Autodesk Fusion 360 part; units mm, degrees
note: some values were not read from the file. Set by a fixed rule: which face or edge a step refers to.
(part 2 of 2)
sketch "Sketch1 (3)" plane through (-20, 0, 0) normal (-1, 0, 0) x (0, -1, 0) in component "Brazo_superior"
  spline S0 degree 5 poles (211.9586, 262.8712) (213.9, 262.5) (215, 260) (215, 257) (212.5679, 252.5298) (212.2678, 249.9329) (212.5261, 247.5635) (214.6128, 241.6791) (217, 240) (218.5775, 235.2522) (220, 231) (221, 229) (220.5807, 226.196) (217.5759, 223.692) (213.5278, 221.7305) (209.5631, 220.0194) (204.555, 219.2265) (203, 220) (201.592, 223.2329) (202, 228) (201.9676, 233.4159) (203.5534, 240.5523) (204.8472, 246.5619) (206.5583, 254.533) (209.5, 263.2) (210.4715, 262.8927) (211.9586, 262.8712) knots 0 0 0 0 0 0 0.045455 0.090909 0.136364 0.181818 0.227273 0.272727 0.318182 0.363636 0.409091 0.454545 0.5 0.545455 0.590909 0.636364 0.681818 0.727273 0.772727 0.818182 0.863636 0.909091 0.954545 1 1 1 1 1 1
  spline S1 degree 5 poles (261, 320) (260.7774, 319.9589) (260.296, 319.9643) (259.4625, 320.2428) (258.1325, 321.1584) (256.169, 323.121) (254.0011, 325.7467) (251.739, 328.8478) (249.4883, 332.2331) (247.3274, 335.7454) (245.3055, 339.2672) (243.4488, 342.7117) (241.7644, 346.0192) (240.2451, 349.1514) (238.8737, 352.0857) (237.6281, 354.8109) (236.4846, 357.3206) (235.4258, 359.6112) (234.4564, 361.6897) (233.6206, 363.5797) (233.0136, 365.3267) (232.8084, 367.0089) (233.2246, 368.7247) (234.4249, 370.5487) (236.4437, 372.5039) (239.0716, 374.5107) (241.9507, 376.4378) (244.6888, 378.1513) (247.0272, 379.6106) (248.853, 380.8435) (250.59, 382.2095) (252.6141, 383.9228) (254.5082, 385.553) (255.9404, 386.771) (256.8623, 387.5494) (258.3073, 388.9023) (260.3731, 390.8134) (262.725, 392.7952) (264.822, 394.1558) (266.2188, 394.3429) (266.8921, 393.3204) (267.1118, 391.4187) (267.1481, 388.996) (267.134, 386.2763) (267.1221, 383.4019) (267.1026, 380.4443) (267.0374, 377.4316) (266.8857, 374.368) (266.6365, 371.2585) (266.3041, 368.1107) (265.9189, 364.9337) (265.5197, 361.7382) (265.1452, 358.5361) (264.827, 355.3399) (264.5793, 352.1629) (264.3983, 349.0181) (264.2687, 345.918) (264.1682, 342.8735) (264.0738, 339.8935) (263.9654, 336.984) (263.8335, 334.147) (263.6787, 331.3832) (263.501, 328.7082) (263.2907, 326.1645) (263.0185, 323.8353) (262.6258, 321.8583) (262.1382, 320.7217) (261.6314, 320.2111) (261.2226, 320.0411) (261, 320) knots 0 0 0 0 0 0 0.01538462 0.03076923 0.04615385 0.06153846 0.07692308 0.09230769 0.10769231 0.12307692 0.13846154 0.15384615 0.16923077 0.18461538 0.2 0.21538462 0.23076923 0.24615385 0.26153846 0.27692308 0.29230769 0.30769231 0.32307692 0.33846154 0.35384615 0.36923077 0.38461538 0.4 0.41538462 0.43076923 0.44615385 0.46153846 0.47692308 0.49230769 0.50769231 0.52307692 0.53846154 0.55384615 0.56923077 0.58461538 0.6 0.61538462 0.63076923 0.64615385 0.66153846 0.67692308 0.69230769 0.70769231 0.72307692 0.73846154 0.75384615 0.76923077 0.78461538 0.8 0.81538462 0.83076923 0.84615385 0.86153846 0.87692308 0.89230769 0.90769231 0.92307692 0.93846154 0.95384615 0.96923077 0.98461538 1 1 1 1 1 1
  spline S2 degree 5 poles (213.7541, 291.5012) (213.7836, 292.1337) (213.9165, 293.5506) (214.3357, 296.1342) (215.3059, 300.4504) (217.0551, 306.9808) (219.1416, 314.1905) (221.3444, 321.5493) (223.447, 328.5165) (225.2663, 334.6064) (226.678, 339.4493) (227.6481, 342.8655) (228.2526, 344.9081) (228.7265, 345.9852) (229.415, 346.7173) (230.5211, 347.2402) (231.9417, 346.7519) (233.4976, 344.3536) (235.4615, 340.7393) (237.9174, 336.5993) (240.7362, 332.3678) (243.6759, 328.3703) (246.4235, 324.7873) (248.6618, 321.698) (250.1239, 319.0883) (250.6571, 316.8737) (250.2721, 314.9163) (249.0801, 313.0601) (247.2465, 311.16) (244.9297, 309.119) (242.2549, 306.9017) (239.3271, 304.5172) (236.2338, 302.0107) (233.052, 299.4513) (229.8531, 296.9221) (226.7094, 294.5083) (223.6983, 292.2901) (220.9029, 290.3618) (218.4131, 288.8445) (216.3267, 287.9051) (214.7483, 287.7655) (213.986, 288.5405) (213.7397, 289.7559) (213.7247, 290.8688) (213.7541, 291.5012) knots 0 0 0 0 0 0 0.025 0.05 0.075 0.1 0.125 0.15 0.175 0.2 0.225 0.25 0.275 0.3 0.325 0.35 0.375 0.4 0.425 0.45 0.475 0.5 0.525 0.55 0.575 0.6 0.625 0.65 0.675 0.7 0.725 0.75 0.775 0.8 0.825 0.85 0.875 0.9 0.925 0.95 0.975 1 1 1 1 1 1
  spline S3 degree 5 poles (213.9418, 208.154) (213.814, 207.7824) (213.413, 207.0453) (212.3788, 205.9701) (210.2085, 204.6435) (206.5692, 203.2643) (202.5179, 202.2474) (198.6058, 201.6547) (195.339, 201.5236) (193.0886, 201.8616) (192.0173, 202.6437) (191.9595, 203.8037) (192.5257, 205.2474) (193.2802, 206.8702) (193.9221, 208.5769) (194.3624, 210.2884) (194.6519, 211.9313) (194.9497, 213.4312) (195.4767, 214.7047) (196.4747, 215.6545) (198.1353, 216.19) (200.5393, 216.2433) (203.5777, 215.7898) (206.9221, 214.8595) (210.1263, 213.5214) (212.7024, 211.8749) (213.9048, 210.4054) (214.1797, 209.275) (214.0696, 208.5256) (213.9418, 208.154) knots -1 -1 -1 -1 -1 -1 -0.96 -0.92 -0.88 -0.84 -0.8 -0.76 -0.72 -0.68 -0.64 -0.6 -0.56 -0.52 -0.48 -0.44 -0.4 -0.36 -0.32 -0.28 -0.24 -0.2 -0.16 -0.12 -0.08 -0.04 0 0 0 0 0 0
  spline S4 degree 3 poles (231.4249, 227.1643) (225.7976, 239.2027) (227.1439, 245.9013) (243.6188, 239.3572) knots -0.949588 -0.949588 -0.949588 -0.949588 -0.175444 -0.175444 -0.175444 -0.175444
  arc A0 (243.9542, 237.7182) -> (243.6188, 239.3572) centre (243.2497, 238.4278) ccw
  line L0 (243.9542, 237.7182) -> (233.0354, 226.8781)
  arc A1 (231.4249, 227.1643) -> (233.0354, 226.8781) centre (232.3308, 227.5878) ccw
  spline S5 degree 5 poles (231.7906, 374.6038) (231.4727, 374.6867) (230.9436, 374.9872) (230.4758, 375.8505) (230.4896, 377.828) (231.4057, 381.5458) (232.9697, 386.2702) (234.8887, 391.6809) (236.8701, 397.4028) (238.6668, 403.0322) (240.1185, 408.1637) (241.201, 412.4145) (242.0021, 415.4706) (242.6867, 417.1356) (243.4659, 417.3808) (244.5652, 416.391) (246.1926, 414.6246) (248.4842, 412.6799) (251.4272, 411.1358) (254.8307, 410.4192) (258.172, 410.6183) (261.1969, 411.5005) (263.7992, 412.6594) (265.9511, 413.6215) (267.6286, 413.9612) (268.7121, 413.4336) (269.0428, 412) (268.6144, 409.8039) (267.6058, 407.1298) (266.2667, 404.3068) (264.8371, 401.6282) (263.455, 399.2654) (262.0644, 397.18) (260.4872, 395.1985) (258.5019, 393.0953) (255.9201, 390.6713) (252.6635, 387.8353) (248.8407, 384.6832) (244.694, 381.4466) (240.548, 378.4434) (236.7582, 376.0277) (234.2798, 374.8383) (232.851, 374.4896) (232.1085, 374.5208) (231.7906, 374.6038) knots -1 -1 -1 -1 -1 -1 -0.975 -0.95 -0.925 -0.9 -0.875 -0.85 -0.825 -0.8 -0.775 -0.75 -0.725 -0.7 -0.675 -0.65 -0.625 -0.6 -0.575 -0.55 -0.525 -0.5 -0.475 -0.45 -0.425 -0.4 -0.375 -0.35 -0.325 -0.3 -0.275 -0.25 -0.225 -0.2 -0.175 -0.15 -0.125 -0.1 -0.075 -0.05 -0.025 0 0 0 0 0 0
  spline S6 degree 5 poles (227.3096, 258.9797) (226.9432, 259.1978) (226.2016, 259.7451) (225.0348, 260.8843) (223.2769, 262.8723) (220.9461, 265.8348) (218.8092, 268.9034) (217.2191, 271.7616) (216.4409, 274.1709) (216.3575, 275.9607) (216.9709, 277.3411) (218.3999, 278.723) (220.7214, 280.4961) (223.8779, 282.8245) (227.7009, 285.6855) (231.9484, 288.9151) (236.3362, 292.2511) (240.5719, 295.3758) (244.387, 297.9591) (247.5704, 299.7014) (250.0012, 300.3759) (251.6838, 299.8733) (252.7099, 298.1966) (253.2192, 295.4532) (253.3561, 291.8523) (253.2502, 287.6795) (253.0108, 283.2567) (252.7167, 278.9076) (252.4087, 274.921) (252.0792, 271.5133) (251.6662, 268.796) (251.0366, 266.7268) (250.0265, 265.154) (248.5043, 263.8975) (246.4235, 262.8169) (243.8891, 261.8877) (241.1096, 261.1639) (238.3081, 260.6365) (235.6845, 260.2815) (233.2736, 259.6803) (231.0644, 258.7491) (229.4862, 258.2952) (228.3997, 258.4361) (227.6759, 258.7615) (227.3096, 258.9797) knots 0 0 0 0 0 0 0.025 0.05 0.075 0.1 0.125 0.15 0.175 0.2 0.225 0.25 0.275 0.3 0.325 0.35 0.375 0.4 0.425 0.45 0.475 0.5 0.525 0.55 0.575 0.6 0.625 0.65 0.675 0.7 0.725 0.75 0.775 0.8 0.825 0.85 0.875 0.9 0.925 0.95 0.975 1 1 1 1 1 1
  spline S7 degree 5 poles (183, 198) (182.8217, 198.0165) (182.557, 198.2746) (182.4163, 199.3066) (182.5436, 201.685) (182.4662, 205.1979) (181.4757, 208.1349) (179.2884, 209.7746) (176.4408, 210.3) (173.9796, 210.4944) (172.9787, 211.2465) (174.0981, 213.105) (177.1726, 215.8633) (181.5132, 218.8579) (186.1365, 221.1984) (190.0241, 222.0271) (192.3467, 220.7457) (192.7517, 217.3103) (191.4825, 212.3413) (189.1238, 206.8171) (186.4319, 201.8613) (184.5946, 199.1691) (183.6268, 198.1755) (183.1783, 197.9835) (183, 198) knots 0 0 0 0 0 0 0.05 0.1 0.15 0.2 0.25 0.3 0.35 0.4 0.45 0.5 0.55 0.6 0.65 0.7 0.75 0.8 0.85 0.9 0.95 1 1 1 1 1 1
  circle A2 centre (223.3374, 249.0861) radius 8.5
  circle A3 centre (176.4838, 204.0852) radius 5
  line L1 (189.4633, 232.5912) -> (169.1821, 210.9178)
  arc A4 (169.1821, 210.9178) -> (178.7602, 194.3477) centre (176.4838, 204.0852) ccw
  line L2 (178.7602, 194.3477) -> (215.6605, 202.9742)
  arc A5 (215.6605, 202.9742) -> (226.6871, 209.9081) centre (211.1076, 222.4491) ccw
  line L3 (226.6871, 209.9081) -> (256.5218, 246.971)
  arc A6 (256.5218, 246.971) -> (260.8937, 258.1191) centre (240.9423, 259.5121) ccw
  line L4 (260.8937, 258.1191) -> (273.342, 436.4099)
  arc A7 (273.342, 436.4099) -> (243.8201, 441.0681) centre (258.3784, 437.4547) ccw
  line L5 (243.8201, 441.0681) -> (194.2709, 241.4386)
  arc A8 (189.4633, 232.5912) -> (194.2709, 241.4386) centre (174.8599, 246.2565) ccw
  spline S8 degree 5 poles (211.9586, 262.8712) (210.4715, 262.8927) (209.5, 263.2) (206.5583, 254.533) (204.8472, 246.5619) (203.5534, 240.5523) (201.9676, 233.4159) (202, 228) (201.592, 223.2329) (203, 220) (204.555, 219.2265) (209.5631, 220.0194) (213.5278, 221.7305) (217.5759, 223.692) (220.5807, 226.196) (221, 229) (220, 231) (218.5775, 235.2522) (217, 240) (214.6128, 241.6791) (212.5261, 247.5635) (212.2678, 249.9329) (212.5679, 252.5298) (215, 257) (215, 260) (213.9, 262.5) (211.9586, 262.8712) knots -1 -1 -1 -1 -1 -1 -0.954545 -0.909091 -0.863636 -0.818182 -0.772727 -0.727273 -0.681818 -0.636364 -0.590909 -0.545455 -0.5 -0.454545 -0.409091 -0.363636 -0.318182 -0.272727 -0.227273 -0.181818 -0.136364 -0.090909 -0.045455 0 0 0 0 0 0
  spline S9 degree 5 poles (261, 320) (261.2226, 320.0411) (261.6314, 320.2111) (262.1382, 320.7217) (262.6258, 321.8583) (263.0185, 323.8353) (263.2907, 326.1645) (263.501, 328.7082) (263.6787, 331.3832) (263.8335, 334.147) (263.9654, 336.984) (264.0738, 339.8935) (264.1682, 342.8735) (264.2687, 345.918) (264.3983, 349.0181) (264.5793, 352.1629) (264.827, 355.3399) (265.1452, 358.5361) (265.5197, 361.7382) (265.9189, 364.9337) (266.3041, 368.1107) (266.6365, 371.2585) (266.8857, 374.368) (267.0374, 377.4316) (267.1026, 380.4443) (267.1221, 383.4019) (267.134, 386.2763) (267.1481, 388.996) (267.1118, 391.4187) (266.8921, 393.3204) (266.2188, 394.3429) (264.822, 394.1558) (262.725, 392.7952) (260.3731, 390.8134) (258.3073, 388.9023) (256.8623, 387.5494) (255.9404, 386.771) (254.5082, 385.553) (252.6141, 383.9228) (250.59, 382.2095) (248.853, 380.8435) (247.0272, 379.6106) (244.6888, 378.1513) (241.9507, 376.4378) (239.0716, 374.5107) (236.4437, 372.5039) (234.4249, 370.5487) (233.2246, 368.7247) (232.8084, 367.0089) (233.0136, 365.3267) (233.6206, 363.5797) (234.4564, 361.6897) (235.4258, 359.6112) (236.4846, 357.3206) (237.6281, 354.8109) (238.8737, 352.0857) (240.2451, 349.1514) (241.7644, 346.0192) (243.4488, 342.7117) (245.3055, 339.2672) (247.3274, 335.7454) (249.4883, 332.2331) (251.739, 328.8478) (254.0011, 325.7467) (256.169, 323.121) (258.1325, 321.1584) (259.4625, 320.2428) (260.296, 319.9643) (260.7774, 319.9589) (261, 320) knots -1 -1 -1 -1 -1 -1 -0.98461538 -0.96923077 -0.95384615 -0.93846154 -0.92307692 -0.90769231 -0.89230769 -0.87692308 -0.86153846 -0.84615385 -0.83076923 -0.81538462 -0.8 -0.78461538 -0.76923077 -0.75384615 -0.73846154 -0.72307692 -0.70769231 -0.69230769 -0.67692308 -0.66153846 -0.64615385 -0.63076923 -0.61538462 -0.6 -0.58461538 -0.56923077 -0.55384615 -0.53846154 -0.52307692 -0.50769231 -0.49230769 -0.47692308 -0.46153846 -0.44615385 -0.43076923 -0.41538462 -0.4 -0.38461538 -0.36923077 -0.35384615 -0.33846154 -0.32307692 -0.30769231 -0.29230769 -0.27692308 -0.26153846 -0.24615385 -0.23076923 -0.21538462 -0.2 -0.18461538 -0.16923077 -0.15384615 -0.13846154 -0.12307692 -0.10769231 -0.09230769 -0.07692308 -0.06153846 -0.04615385 -0.03076923 -0.01538462 0 0 0 0 0 0
  spline S10 degree 5 poles (213.7541, 291.5012) (213.7247, 290.8688) (213.7397, 289.7559) (213.986, 288.5405) (214.7483, 287.7655) (216.3267, 287.9051) (218.4131, 288.8445) (220.9029, 290.3618) (223.6983, 292.2901) (226.7094, 294.5083) (229.8531, 296.9221) (233.052, 299.4513) (236.2338, 302.0107) (239.3271, 304.5172) (242.2549, 306.9017) (244.9297, 309.119) (247.2465, 311.16) (249.0801, 313.0601) (250.2721, 314.9163) (250.6571, 316.8737) (250.1239, 319.0883) (248.6618, 321.698) (246.4235, 324.7873) (243.6759, 328.3703) (240.7362, 332.3678) (237.9174, 336.5993) (235.4615, 340.7393) (233.4976, 344.3536) (231.9417, 346.7519) (230.5211, 347.2402) (229.415, 346.7173) (228.7265, 345.9852) (228.2526, 344.9081) (227.6481, 342.8655) (226.678, 339.4493) (225.2663, 334.6064) (223.447, 328.5165) (221.3444, 321.5493) (219.1416, 314.1905) (217.0551, 306.9808) (215.3059, 300.4504) (214.3357, 296.1342) (213.9165, 293.5506) (213.7836, 292.1337) (213.7541, 291.5012) knots -1 -1 -1 -1 -1 -1 -0.975 -0.95 -0.925 -0.9 -0.875 -0.85 -0.825 -0.8 -0.775 -0.75 -0.725 -0.7 -0.675 -0.65 -0.625 -0.6 -0.575 -0.55 -0.525 -0.5 -0.475 -0.45 -0.425 -0.4 -0.375 -0.35 -0.325 -0.3 -0.275 -0.25 -0.225 -0.2 -0.175 -0.15 -0.125 -0.1 -0.075 -0.05 -0.025 0 0 0 0 0 0
  spline S11 degree 5 poles (213.9418, 208.154) (214.0696, 208.5256) (214.1797, 209.275) (213.9048, 210.4054) (212.7024, 211.8749) (210.1263, 213.5214) (206.9221, 214.8595) (203.5777, 215.7898) (200.5393, 216.2433) (198.1353, 216.19) (196.4747, 215.6545) (195.4767, 214.7047) (194.9497, 213.4312) (194.6519, 211.9313) (194.3624, 210.2884) (193.9221, 208.5769) (193.2802, 206.8702) (192.5257, 205.2474) (191.9595, 203.8037) (192.0173, 202.6437) (193.0886, 201.8616) (195.339, 201.5236) (198.6058, 201.6547) (202.5179, 202.2474) (206.5692, 203.2643) (210.2085, 204.6435) (212.3788, 205.9701) (213.413, 207.0453) (213.814, 207.7824) (213.9418, 208.154) knots 0 0 0 0 0 0 0.04 0.08 0.12 0.16 0.2 0.24 0.28 0.32 0.36 0.4 0.44 0.48 0.52 0.56 0.6 0.64 0.68 0.72 0.76 0.8 0.84 0.88 0.92 0.96 1 1 1 1 1 1
  spline S12 degree 3 poles (243.6188, 239.3572) (227.1439, 245.9013) (225.7976, 239.2027) (231.4249, 227.1643) knots 0.175444 0.175444 0.175444 0.175444 0.949588 0.949588 0.949588 0.949588
  arc A9 (231.4249, 227.1643) -> (233.0354, 226.8781) centre (232.3308, 227.5878) ccw
  line L6 (233.0354, 226.8781) -> (243.9542, 237.7182)
  arc A10 (243.9542, 237.7182) -> (243.6188, 239.3572) centre (243.2497, 238.4278) ccw
  spline S13 degree 5 poles (231.7906, 374.6038) (232.1085, 374.5208) (232.851, 374.4896) (234.2798, 374.8383) (236.7582, 376.0277) (240.548, 378.4434) (244.694, 381.4466) (248.8407, 384.6832) (252.6635, 387.8353) (255.9201, 390.6713) (258.5019, 393.0953) (260.4872, 395.1985) (262.0644, 397.18) (263.455, 399.2654) (264.8371, 401.6282) (266.2667, 404.3068) (267.6058, 407.1298) (268.6144, 409.8039) (269.0428, 412) (268.7121, 413.4336) (267.6286, 413.9612) (265.9511, 413.6215) (263.7992, 412.6594) (261.1969, 411.5005) (258.172, 410.6183) (254.8307, 410.4192) (251.4272, 411.1358) (248.4842, 412.6799) (246.1926, 414.6246) (244.5652, 416.391) (243.4659, 417.3808) (242.6867, 417.1356) (242.0021, 415.4706) (241.201, 412.4145) (240.1185, 408.1637) (238.6668, 403.0322) (236.8701, 397.4028) (234.8887, 391.6809) (232.9697, 386.2702) (231.4057, 381.5458) (230.4896, 377.828) (230.4758, 375.8505) (230.9436, 374.9872) (231.4727, 374.6867) (231.7906, 374.6038) knots 0 0 0 0 0 0 0.025 0.05 0.075 0.1 0.125 0.15 0.175 0.2 0.225 0.25 0.275 0.3 0.325 0.35 0.375 0.4 0.425 0.45 0.475 0.5 0.525 0.55 0.575 0.6 0.625 0.65 0.675 0.7 0.725 0.75 0.775 0.8 0.825 0.85 0.875 0.9 0.925 0.95 0.975 1 1 1 1 1 1
  spline S14 degree 5 poles (227.3096, 258.9797) (227.6759, 258.7615) (228.3997, 258.4361) (229.4862, 258.2952) (231.0644, 258.7491) (233.2736, 259.6803) (235.6845, 260.2815) (238.3081, 260.6365) (241.1096, 261.1639) (243.8891, 261.8877) (246.4235, 262.8169) (248.5043, 263.8975) (250.0265, 265.154) (251.0366, 266.7268) (251.6662, 268.796) (252.0792, 271.5133) (252.4087, 274.921) (252.7167, 278.9076) (253.0108, 283.2567) (253.2502, 287.6795) (253.3561, 291.8523) (253.2192, 295.4532) (252.7099, 298.1966) (251.6838, 299.8733) (250.0012, 300.3759) (247.5704, 299.7014) (244.387, 297.9591) (240.5719, 295.3758) (236.3362, 292.2511) (231.9484, 288.9151) (227.7009, 285.6855) (223.8779, 282.8245) (220.7214, 280.4961) (218.3999, 278.723) (216.9709, 277.3411) (216.3575, 275.9607) (216.4409, 274.1709) (217.2191, 271.7616) (218.8092, 268.9034) (220.9461, 265.8348) (223.2769, 262.8723) (225.0348, 260.8843) (226.2016, 259.7451) (226.9432, 259.1978) (227.3096, 258.9797) knots -1 -1 -1 -1 -1 -1 -0.975 -0.95 -0.925 -0.9 -0.875 -0.85 -0.825 -0.8 -0.775 -0.75 -0.725 -0.7 -0.675 -0.65 -0.625 -0.6 -0.575 -0.55 -0.525 -0.5 -0.475 -0.45 -0.425 -0.4 -0.375 -0.35 -0.325 -0.3 -0.275 -0.25 -0.225 -0.2 -0.175 -0.15 -0.125 -0.1 -0.075 -0.05 -0.025 0 0 0 0 0 0
  spline S15 degree 5 poles (183, 198) (183.1783, 197.9835) (183.6268, 198.1755) (184.5946, 199.1691) (186.4319, 201.8613) (189.1238, 206.8171) (191.4825, 212.3413) (192.7517, 217.3103) (192.3467, 220.7457) (190.0241, 222.0271) (186.1365, 221.1984) (181.5132, 218.8579) (177.1726, 215.8633) (174.0981, 213.105) (172.9787, 211.2465) (173.9796, 210.4944) (176.4408, 210.3) (179.2884, 209.7746) (181.4757, 208.1349) (182.4662, 205.1979) (182.5436, 201.685) (182.4163, 199.3066) (182.557, 198.2746) (182.8217, 198.0165) (183, 198) knots -1 -1 -1 -1 -1 -1 -0.95 -0.9 -0.85 -0.8 -0.75 -0.7 -0.65 -0.6 -0.55 -0.5 -0.45 -0.4 -0.35 -0.3 -0.25 -0.2 -0.15 -0.1 -0.05 0 0 0 0 0 0
  circle A11 centre (223.3374, 249.0861) radius 8.5
  circle A12 centre (176.4838, 204.0852) radius 5
  line L7 (169.1821, 210.9178) -> (189.4633, 232.5912)
  arc A13 (189.4633, 232.5912) -> (194.2709, 241.4386) centre (174.8599, 246.2565) ccw
  line L8 (194.2709, 241.4386) -> (243.8201, 441.0681)
  arc A14 (273.342, 436.4099) -> (243.8201, 441.0681) centre (258.3784, 437.4547) ccw
  line L9 (273.342, 436.4099) -> (260.8937, 258.1191)
  arc A15 (256.5218, 246.971) -> (260.8937, 258.1191) centre (240.9423, 259.5121) ccw
  line L10 (256.5218, 246.971) -> (226.6871, 209.9081)
  arc A16 (215.6605, 202.9742) -> (226.6871, 209.9081) centre (211.1076, 222.4491) ccw
  line L11 (215.6605, 202.9742) -> (178.7602, 194.3477)
  arc A17 (169.1821, 210.9178) -> (178.7602, 194.3477) centre (176.4838, 204.0852) ccw
  circle A18 centre (251.5224, 254.8379) radius 5
  circle A19 centre (210.2447, 276.6455) radius 5
  circle A20 centre (229.886, 355.7504) radius 5
  line L12 (240.9423, 259.5121) -> (267, 248) construction
  line L13 (211.9586, 262.8712) -> (220.2942, 266.8312) construction
  line L14 (223.3374, 249.0861) -> (202, 294) construction
  circle A21 centre (257.7483, 430.3868) radius 12.5
  dimension "d277" = 10
  dimension "d278" = 10
  dimension "d279" = 10
  dimension "d282" = 25
  constraint coincident A6.centre A15.centre
  constraint coincident A18.centre L12
  constraint coincident S0.start S0.end
  constraint coincident S14 L13.end
  constraint coincident S6 L13.end
  constraint coincident A2.centre A11.centre
  constraint perpendicular L13 L14
  constraint coincident A19.centre L14
  measures "d277" diameter of A18
  measures "d278" diameter of A19
  measures "d279" diameter of A20
  measures "d282" diameter of A21
extrude "Extrude3'" add sketch "Sketch1 (3)" along normal up to surface (120 mm away) contours A18 | A19 | A20 bodies 7 in component "Brazo_superior"
extrude "Extrude4''" cut sketch "Sketch1 (3)" along normal through all and the other way through all contours A21 bodies 7 in component "Brazo_superior"
component "Brazo_inferior" placed x (1, 0, 0) y (0, 1, 0) z (0, 0, 1) at (0, 0, 0)
component "Base" placed x (1, 0, 0) y (0, 1, 0) z (0, 0, 1) at (0, 0, 0)
component "Brazo_superior" placed x (1, 0, 0) y (0, 1, 0) z (0, 0, 1) at (0, 0, 0)
component "Axis_slider_crank" placed x (1, 0, 0) y (0, 1, 0) z (0, 0, 1) at (0, 0, 0)
component "SliderUp" placed x (1, 0, 0) y (0, 1, 0) z (0, 0, 1) at (0, 0, 0)
component "SliderBot" placed x (1, 0, 0) y (0, 1, 0) z (0, 0, 1) at (0, 0, 0)
component "Crank" placed x (1, 0, 0) y (0, 1, 0) z (0, 0, 1) at (0, 0, 0)
hidden bodies 3
named bodies: "Base", "Brazo_inferior", "Brazo_superior", "SliderUp", "SliderBot", "Axis_slider_crank", "Crank", "Brazo_inferior (1)", "Brazo_superior (1)"
